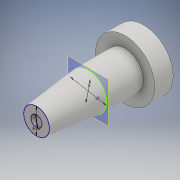
# Autodesk Inventor part: vacuum-nozzle-shaft
Saved by Autodesk Inventor 2017 (Build 210142000, 142)
## iProperties
Created: 2026-03-25
Part Number: vacuum-nozzle-shaft
Material: Generic
Document SubType Name: Modeling
Designer: a
Density: 1 g/cm^3
Appearance: Default
Author: a
Autodesk Inventor part; units mm, degrees
ref_plane "YZ Plane" through (0, 0, 0) normal (1, 0, 0) x (0, 1, 0)
ref_plane "XY Plane" through (0, 0, 0) normal (0, 0, 1) x (1, 0, 0)
sketch "Sketch1" plane through (0, 0, 0) normal (0, 1, 0) x (-1, 0, 0)
  circle A0 centre (0, 0) radius 3.475
  circle A1 centre (0, 0) radius 1.5
  dimension "d0" = 6.95
  dimension "d11" = 3
  constraints: 2 centre point, 2 coincident
  measures "d0" diameter of A0
  measures "d11" diameter of A1
ref_plane "Work Plane1" through (0, 14, 0) normal (0, 1, 0) x (-1, 0, 0)
sketch "Sketch2" plane through (0, 14, 0) normal (0, 1, 0) x (-1, 0, 0)
  circle A0 centre (0, 0) radius 5
  circle A1 centre (0, 0) radius 3
  dimension "d6" = 10
  dimension "d12" = 6
  constraints: 2 centre point, 1 coincident
  measures "d6" diameter of A0
  measures "d12" diameter of A1
loft "Loft1" add profiles "Sketch1", "Sketch2" contours A0 | A1 / A0 | A1
extrude "Extrusion2" add sketch "Sketch2" along normal blind 10
hole "Hole3" at (0, 0, 0) direction (0, 1, 0) diameter 3 end through all
loft "Loft2" cut section 1 edges at (0, 0, 1.5) section 2 edges at (3, 14, 0)
sketch "Sketch3" plane through (0, 24, 0) normal (0, 1, 0) x (1, 0, 0)
  circle A0 centre (0, 0) radius 3
  circle A1 centre (0, 0) radius 5.1
  circle A2 centre (0, 0) radius 1.5 projected
  line L0 (0, 5.1) -> (4.4167, 2.55)
  line L1 (4.4167, 2.55) -> (4.4167, -2.55)
  line L2 (4.4167, -2.55) -> (0, -5.1)
  line L3 (0, -5.1) -> (-4.4167, -2.55)
  line L4 (-4.4167, -2.55) -> (-4.4167, 2.55)
  line L5 (-4.4167, 2.55) -> (0, 5.1)
  circle A3 centre (0, 0) radius 8
  dimension "d43" = 10.2
  dimension "d42" = 6
  dimension "d44" = 16
  constraints: 12 end point, 4 coincident, 2 centre point, 1 vertical alignment, 15 other
  measures "d42" diameter of A0
  measures "d44" diameter of A3
extrude "Extrusion3" add sketch "Sketch3" along normal blind 5 contours A1 L1 | L0 A1 | A1 L2 | L5 A1 | A1 L3 | L4 A1 | A3
body "Solid1"
